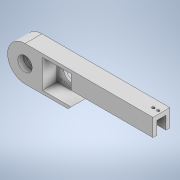
# Autodesk Inventor part: force_measurement_thingy
Saved by Autodesk Inventor 2022 (Build 260153000, 153)
## iProperties
Created: 2022-01-28
Part Number: force_measurement_thingy
Material: Generic
Document SubType Name: Modeling
Designer: Martijn
Density: 1 g/cm^3
Appearance: Default
Author: Martijn
Autodesk Inventor part; units mm, degrees
ref_plane "YZ Plane" through (0, 0, 0) normal (1, 0, 0) x (0, 1, 0)
ref_plane "XZ Plane" through (0, 0, 0) normal (0, 1, 0) x (-1, 0, 0)
ref_plane "XY Plane" through (0, 0, 0) normal (0, 0, 1) x (1, 0, 0)
sketch "Sketch1" plane through (0, 0, 0) normal (0, 0, 1) x (1, 0, 0)
  arc A0 (0, 27) -> (0, -27) centre (0, 0) ccw
  line L0 (0, 27) -> (71, 27)
  line L1 (71, 27) -> (71, -27)
  line L2 (71, -27) -> (0, -27)
  dimension "d0" = 27
  dimension "d2" = 71
  constraints: 6 end point, 2 perpendicular, 2 point on circle, 1 centre point, 1 coincident, 1 horizontal, 1 tangent
  measures "d0" radius of A0
  measures "d2" distance from line of point (0, 0) L1
extrude "Extrusion1" add sketch "Sketch1" against normal blind 26
sketch "Sketch2" plane through (0, 0, 0) normal (0, 0, 1) x (1, 0, 0)
  circle A0 centre (0, 0) radius 11
  dimension "d5" = 22
  constraints: 1 centre point, 1 coincident
  measures "d5" diameter of A0
extrude "Extrusion2" cut sketch "Sketch2" against normal blind 8
sketch "Sketch3" plane through (0, 0, -26) normal (0, 0, -1) x (-1, 0, 0)
  circle A0 centre (0, 0) radius 11 projected
  circle A1 centre (0, 0) radius 11
  dimension "d8" = 22
  constraints: 1 centre point, 1 coincident
  measures "d8" diameter of A1
extrude "Extrusion3" cut sketch "Sketch3" against normal blind 8
sketch "Sketch4" plane through (0, 0, -26) normal (0, 0, -1) x (-1, 0, 0)
  line L0 (-27, 22) -> (-27, -22)
  line L1 (-27, -22) -> (-71, -22)
  line L2 (-71, -22) -> (-71, 22)
  line L3 (-71, 22) -> (-27, 22)
  line L4 (0, 27) -> (-71, 27) projected
  line L5 (-71, 27) -> (-71, -27) projected
  point P0 (0, 0)
  dimension "d11" = 44
  dimension "d18" = 44
  dimension "d19" = 5
  constraints: 8 end point, 2 parallel, 1 collinear, 1 vertical
  measures "d11" distance between parallel lines of L2 L0
  measures "d18" distance between parallel lines of L1 L3
  measures "d19" distance between parallel lines of L3 L4
extrude "Extrusion4" cut sketch "Sketch4" against normal blind 22
sketch "Sketch5" plane through (0, 0, -4) normal (0, 0, -1) x (-1, 0, 0)
  circle A0 centre (-49, 0) radius 11.5
  line L0 (-71, -22) -> (-71, 22) projected
  line L1 (-71, -27) -> (0, -27) projected
  line L2 (-27, -22) -> (-71, -22) projected
  point P0 (0, 0)
  point P1 (-71, 27)
  dimension "d14" = 23
  dimension "d15" = 22
  dimension "d21" = 22
  constraints: 1 centre point
  measures "d14" diameter of A0
  measures "d15" distance from line of L0 A0.centre
  measures "d21" distance from line of L2 A0.centre
extrude "Extrusion5" cut sketch "Sketch5" against normal blind 25
sketch "Sketch6" plane through (0, 0, -4) normal (0, 0, -1) x (-1, 0, 0)
  point P0 (0, 0)
sketch "Sketch7" plane through (0, 0, -4) normal (0, 0, -1) x (-1, 0, 0)
  circle A0 centre (-64.5, 15.5) radius 1.7
  circle A1 centre (-33.5, 15.5) radius 1.7
  circle A2 centre (-33.5, -15.5) radius 1.7
  circle A3 centre (-64.5, -15.5) radius 1.7
  line L0 (-64.5, 15.5) -> (-33.5, 15.5)
  line L1 (-33.5, 15.5) -> (-33.5, -15.5)
  line L2 (-33.5, -15.5) -> (-64.5, -15.5)
  line L3 (-64.5, -15.5) -> (-64.5, 15.5)
  line L4 (-71, -22) -> (-71, 22) projected
  line L5 (-71, 22) -> (-27, 22) projected
  point P0 (0, 0)
  dimension "d22" = 3.4
  dimension "d24" = 31
  dimension "d25" = 31
  dimension "d26" = 6.5
  dimension "d27" = 6.5
  constraints: 8 end point, 4 centre point, 3 equal radius, 3 perpendicular, 1 horizontal
  measures "d22" diameter of A0
  measures "d24" distance of L0.start L0.end
  measures "d25" distance of L1.end L0.end
  measures "d26" distance from line of L4 L2.end
  measures "d27" distance between parallel lines of L0 L5
extrude "Extrusion6" cut sketch "Sketch7" against normal blind 31 contours L0 L3 A0 | A0 L3 L0 | L0 L1 A1 | A1 L1 L0 | L3 L2 A3 | A3 L2 L3 | L1 L2 A2 | A2 L2 L1
sketch "Sketch8" plane through (0, 0, -8) normal (0, 0, 1) x (1, 0, 0)
  circle A0 centre (0, 0) radius 4.3
  dimension "d30" = 8.6
  constraints: 1 centre point, 1 coincident
  measures "d30" diameter of A0
extrude "Extrusion7" cut sketch "Sketch8" against normal blind 30
sketch "Sketch9" plane through (71, -27, 0) normal (1, 0, 0) x (0, 0, -1)
  line L0 (0, 0) -> (0, 54) projected
  line L1 (0, 54) -> (26, 54) projected
  line L2 (26, 54) -> (26, 27)
  line L3 (26, 27) -> (20, 27)
  line L4 (20, 27) -> (20, 49)
  line L5 (20, 49) -> (6, 49)
  line L6 (6, 49) -> (6, 27)
  line L7 (6, 27) -> (0, 27)
  line L8 (0, 54) -> (0, 27)
  line L9 (0, 54) -> (26, 54)
  dimension "d38" = 14
  dimension "d39" = 27
  dimension "d40" = 5
  constraints: 16 end point, 5 perpendicular, 2 collinear, 2 point on line, 1 midpoint, 1 vertical
  measures "d38" distance between parallel lines of L4 L6
  measures "d39" distance between parallel lines of L1 L3
  measures "d40" distance between parallel lines of L1 L5
extrude "Extrusion8" add sketch "Sketch9" along normal blind 126
sketch "Sketch10" plane through (27, 22, -26) normal (0, -1, 0) x (1, 0, 0)
  line L0 (44, 6) -> (170, 6) projected
  line L1 (170, 6) -> (152, 6)
  line L2 (152, 6) -> (152, 20)
  line L3 (152, 20) -> (170, 20)
  line L4 (170, 20) -> (170, 6)
  line L5 (44, 20) -> (170, 20) projected
  line L6 (152, 13) -> (170, 13)
  arc A0 (165.5, 11.3) -> (165.5, 14.7) centre (165.5, 13) ccw
  arc A1 (164.5, 14.7) -> (164.5, 11.3) centre (164.5, 13) ccw
  arc A2 (158, 11.3) -> (158, 14.7) centre (158, 13) ccw
  arc A3 (157, 14.7) -> (157, 11.3) centre (157, 13) ccw
  line L7 (157, 14.7) -> (158, 14.7)
  line L8 (158, 11.3) -> (157, 11.3)
  line L9 (164.5, 14.7) -> (165.5, 14.7)
  line L10 (165.5, 11.3) -> (164.5, 11.3)
  point P0 (-27, 26)
  point P1 (152, 6)
  point P2 (165, 14.7)
  point P3 (157.5, 14.7)
  point P4 (155.3, 13)
  point P5 (159.7, 13)
  point P6 (162.8, 13)
  point P7 (167.2, 13)
  dimension "d41" = 18
  dimension "d59" = 1.7
  dimension "d60" = 1.7
  dimension "d61" = 1
  dimension "d62" = 1
  dimension "d63" = 5
  dimension "d64" = 7.5
  constraints: 18 end point, 8 point on circle, 6 tangent, 5 parallel, 4 centre point, 4 midpoint, 4 point on line, 2 horizontal, 1 collinear, 1 perpendicular
  measures "d41" distance between parallel lines of L4 L2
  measures "d59" radius of A1
  measures "d60" radius of A2
  measures "d61" distance of L9.start L9.end
  measures "d62" distance of L7.start L7.end
  measures "d63" distance from line of L4 point (165, 14.7)
  measures "d64" distance of point (165, 14.7) point (157.5, 14.7)
extrude "Extrusion9" cut sketch "Sketch10" against normal blind 100 contours A3 L7 A2 L6 | L6 A2 L8 A3 | A0 L10 A1 L6 | L6 A1 L9 A0
extrude "Extrusion10" add sketch "Sketch10" along normal blind 2 contours L2 L6 A3 L8 A2 A1 L10 A0 L4 L0 | L2 L3 L4 L6 A0 L9 A1 A2 L7 A3
sketch "Sketch11" plane through (0, 0, 0) normal (0, 0, 1) x (1, 0, 0)
  circle A0 centre (58, -15.5885) radius 1.25
  circle A1 centre (49, 0) radius 11.5 projected
  line L0 (58, -15.5885) -> (49, 0)
  line L1 (71, 0) -> (197, 0) projected
  point P0 (0, 0)
  dimension "d51" = 2.5
  dimension "d52" = 18
  dimension "d53" = 60
  constraints: 2 end point, 1 centre point
  measures "d51" diameter of A0
  measures "d52" distance of L0.end L0.start
  measures "d53" angle of L1 L0
extrude "Extrusion11" cut sketch "Sketch11" against normal blind 10 contours A0
pattern_circular "Circular Pattern1" count 6 over 360 about axis through (49, 0, -4) along (0, 0, 1) of "Extrusion11"
chamfer "Chamfer1" distance 5 angle 45 1 edges at (71, -27, -13)
chamfer "Chamfer2" distance 2 angle 45 4 edges at (35.2, 15.5, 0) (66.2, 15.5, 0) (66.2, -15.5, 0) (35.2, -15.5, 0)
mirror "Mirror1" about plane through (22, 0, 0) normal (0, 0, 1) remove original yes
equation "\"d28\" = d24"
body "Solid1"
